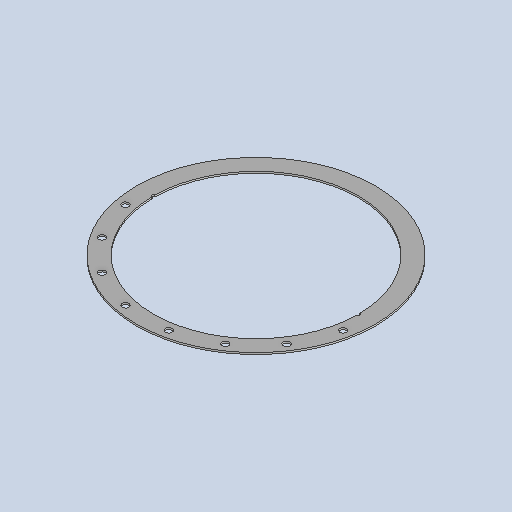
# Autodesk Inventor part: ДМФ 031 кольцо под шпильки НОС v2.0
Saved by Autodesk Inventor 2025 (Build 290162010, 162A)
## iProperties
Created: 2024-04-23
Part Number: ДМФ 031 кольцо под шпильки НОС v2.0
Material: Generic
Document SubType Name: Sheet Metal
Designer: admin
Density: 1 g/cm^3
Appearance: Default
Sheet Metal Rule: Default
Flat Pattern Width: 42 cm
Flat Pattern Length: 42 cm
Flat Pattern Area: 1764 cm^2
Sheet Metal Width: 420,000 mm
Sheet Metal Length: 420,000 mm
Sheet Metal Area: 176400,000 mm^2
Stock Number: ДМС 010 кольцо под шпильки
Author: admin
Autodesk Inventor part; units mm, degrees
note: some values were not read from the file. Chosen so that the rebuilt part matches the saved one: pattern direction of "Circular Pattern1".
ref_plane "YZ Plane" through (0, 0, 0) normal (1, 0, 0) x (0, 1, 0)
ref_plane "XZ Plane" through (0, 0, 0) normal (0, 1, 0) x (-1, 0, 0)
ref_plane "XY Plane" through (0, 0, 0) normal (0, 0, 1) x (1, 0, 0)
sketch "Sketch1" plane through (0, 0, 0) normal (0, 0, 1) x (1, 0, 0)
  circle A0 centre (0, 0) radius 180
  circle A1 centre (0, 0) radius 210
  circle A2 centre (0, 0) radius 195 construction
  line L0 (0, 210) -> (0, 180) construction
  point P0 (0, 195)
  dimension "d9" = 390
  dimension "d11" = 30
extrude "Plate1" add sketch "Sketch1" along normal blind 3
sketch "Sketch2" plane through (0, 0, 3) normal (0, 0, 1) x (1, 0, 0)
  circle A0 centre (0, 0) radius 180 construction
  circle A1 centre (0, 0) radius 210 construction
  circle A2 centre (0, 0) radius 210 projected
  circle A3 centre (0, 0) radius 180 projected
  line L0 (0, 0) -> (0, -210) construction
  line L1 (0, 0) -> (-40.969, -205.9649) construction
  line L2 (-35.1163, -176.5414) -> (-40.969, -205.9649) construction
  circle A4 centre (-38.0426, -191.2531) radius 6
  dimension "d20" = 11.25
  dimension "d21" = 12
  constraints: 6 end point, 2 point on circle, 1 centre point, 1 collinear, 1 midpoint, 1 point on line, 1 vertical, 2 other
  measures "d20" angle of L0 L1
  measures "d21" diameter of A4
extrude "Extrusion1" cut sketch "Sketch2" against normal through all contours A4
pattern_circular "Circular Pattern1" count 8 over 157.5 about axis through (0, 0, 0) along (0, 0, 1) of "Extrusion1" both ways yes
sketch "Sketch3" plane through (0, 0, 3) normal (0, 0, 1) x (1, 0, 0)
  circle A0 centre (0, 0) radius 180 construction
  line L0 (180, 0) -> (-180, 0) construction
  circle A1 centre (180, 0) radius 2.5
  circle A2 centre (-180, 0) radius 2.5
  circle A3 centre (-161.2452, -80) radius 2.5
  line L1 (-161.2452, -80) -> (161.2452, -80) construction
  circle A4 centre (161.2452, -80) radius 2.5
  dimension "d27" = 5
  dimension "d29" = 80
  constraints: 4 centre point, 4 coincident, 4 end point, 4 point on circle, 3 equal radius, 2 horizontal, 1 midpoint
  measures "d27" diameter of A1
  measures "d29" distance between parallel lines of L1 L0
extrude "Extrusion2" cut sketch "Sketch3" against normal through all contours A1 | A2
equation "\"d9\" = Шпил_пласт_НОС_диам_центров"
equation "\"d11\" = Шпил_пласт_НОС_ширина"
equation "\"d21\" = Шпил_пласт_НОС_диам_шпильки"
equation "\"d2\" = Thickness"
equation "\"BendRadius\" = Thickness"
equation "\"BendReliefWidth\" = Thickness"
equation "\"BendReliefDepth\" = 0.5 * Thickness"
equation "\"CornerReliefSize\" = 4 * Thickness"
equation "\"MinimumRemnant\" = 2 * Thickness"
equation "\"TransitionRadius\" = BendRadius"
equation "\"JacobiRadiusSize\" = BendRadius"
equation "\"GapSize\" = Thickness"
equation "\"Шпил_пласт_НОС_диам_центров\" = 390"
equation "\"Шпил_пласт_НОС_ширина\" = 30"
equation "\"Шпил_пласт_НОС_диам_шпильки\" = 12"
equation "\"Thickness\" = 3"
body "Solid1"
